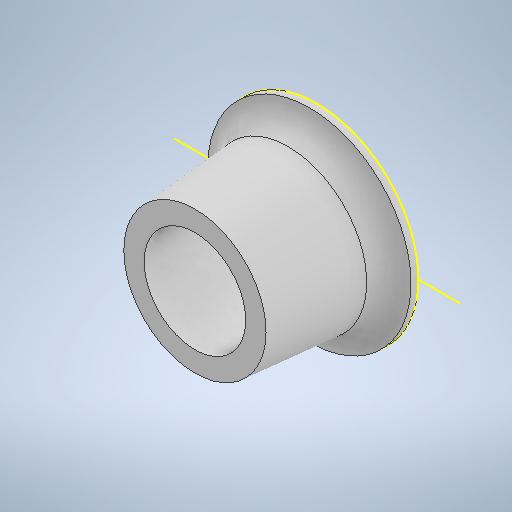
# Autodesk Inventor part: versuch
Saved by Autodesk Inventor 2025.2 (Build 292293000, 293)
## iProperties
Created: 2025-01-31
Part Number: versuch
Material: Generisch
Document SubType Name: Modeling
Designer: unter
Density: 1 g/cm^3
Appearance: Vorgabe
Author: unter
Autodesk Inventor part; units mm, degrees
ref_plane "YZ Plane" through (0, 0, 0) normal (1, 0, 0) x (0, 1, 0)
ref_plane "XZ Plane" through (0, 0, 0) normal (0, 1, 0) x (-1, 0, 0)
ref_plane "XY Plane" through (0, 0, 0) normal (0, 0, 1) x (1, 0, 0)
sketch "Skizze1" plane through (0, 0, 0) normal (1, 0, 0) x (0, 1, 0)
  line L0 (0, 0) -> (-12, 0) construction
  line L1 (0, 10) -> (-0.7247, 10)
  line L2 (-2.8192, 7.7319) -> (-12, 7)
  line L3 (-12, 7) -> (-12, 5)
  line L4 (-12, 5) -> (-4.6713, 5)
  line L5 (-4.6713, 5) -> (-4.6713, 4)
  line L6 (-4.6713, 4) -> (-3.7921, 4)
  line L7 (-3.7921, 4) -> (-3.7921, 2)
  line L8 (-3.7921, 2) -> (0, 2)
  arc A0 (-2.8192, 7.7319) -> (-0.7247, 10) centre (-3, 10) ccw
  line L9 (0, 10) -> (0, 2)
  dimension "d2" = 20
  dimension "d3" = 8
  dimension "d4" = 12
  dimension "d6" = 2
  dimension "d7" = 1
  dimension "d8" = 2
  constraints: 20 end point, 3 perpendicular, 2 horizontal, 2 point on circle, 2 vertical alignment, 1 centre point, 1 parallel, 1 tangent, 1 vertical
  measures "d2" diameter of L1 L0
  measures "d3" distance between parallel lines of L1 L8
  measures "d4" distance between parallel lines of L3 L9
  measures "d6" distance of L6.end L7.end
  measures "d7" distance of L4.end L5.end
  measures "d8" distance of L2.end L3.end
revolve "Umdrehung1" add sketch "Skizze1" angle 360 about axis through (0, 0, 0) along (0, -1, 0)
sketch "Skizze2" plane through (0, 0, 0) normal (0, 1, 0) x (1, 0, 0)
  circle A0 centre (0, 0) radius 10 projected
  circle A1 centre (0, 0) radius 7.7247 projected
  line L0 (-14.0052, 0) -> (14.0309, 0) projected
